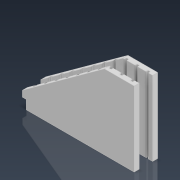
# Autodesk Inventor part: Rising agency
Saved by Autodesk Inventor 2021.1 (Build 251245010, 245A)
## iProperties
Created: 2020-12-20
Part Number: Rising agency
Material: 一般
Document SubType Name: Modeling
Designer: User
Density: 1 g/cm^3
Appearance: 預設
Author: User
Autodesk Inventor part; units mm, degrees
ref_plane "YZ Plane" through (0, 0, 0) normal (1, 0, 0) x (0, 1, 0)
ref_plane "XZ Plane" through (0, 0, 0) normal (0, 1, 0) x (-1, 0, 0)
ref_plane "XY Plane" through (0, 0, 0) normal (0, 0, 1) x (1, 0, 0)
sketch "草圖1" plane through (0, 0, 0) normal (0, 0, 1) x (1, 0, 0)
  line L0 (0, 0) -> (0, 800)
  line L1 (0, 800) -> (-150, 800)
  line L2 (-150, 800) -> (-720, 176.041)
  line L3 (-700, 100) -> (-150, 100)
  line L4 (-150, 100) -> (-150, 0)
  line L5 (-150, 0) -> (0, 0)
  line L6 (-720, 176.041) -> (-720, 146.041)
  line L7 (-720, 146.041) -> (-700, 146.041)
  line L8 (-700, 146.041) -> (-700, 100)
  dimension "d0" = 150
  dimension "d1" = 150
  dimension "d3" = 800
  dimension "d4" = 100
  dimension "d5" = 720
  dimension "d6" = 20
  dimension "d8" = 30
  dimension "d9" = 146.041
  constraints: 18 end point, 5 perpendicular, 2 vertical, 1 horizontal
  measures "d0" distance of L4.end L0.start
  measures "d1" distance of L0.end L1.end
  measures "d3" distance of L0.start L0.end
  measures "d4" distance of L3.end L4.end
  measures "d5" distance between parallel lines of L0 L6
  measures "d6" distance of L6.end L7.end
  measures "d8" distance of L2.end L6.end
  measures "d9" distance between parallel lines of L7 L5
extrude "擠出1" add sketch "草圖1" along normal mid plane 120
sketch "草圖2" plane through (-700, 100, 60) normal (0, -1, 0) x (1, 0, 0)
  line L0 (700, -120) -> (550, -120) construction
  line L1 (550, -120) -> (0, -120) construction
  line L2 (0, -120) -> (0, 0) construction
  line L3 (0, 0) -> (550, 0) construction
  line L4 (550, 0) -> (700, 0) construction
  line L5 (700, 0) -> (700, -120) construction
  line L6 (550, -120) -> (550, 0) construction
  line L7 (-108.104, -26) -> (550, -26)
  line L8 (550, -26) -> (550, -94)
  line L9 (550, -94) -> (-108.104, -94)
  line L10 (-108.104, -94) -> (-108.104, -26)
  point P0 (700, -60)
  point P1 (550, -60)
  dimension "d12" = 68
  constraints: 8 end point, 2 midpoint, 2 parallel, 1 horizontal, 1 perpendicular
  measures "d12" distance of L9.end L7.start
extrude "擠出2" cut sketch "草圖2" against normal through all
sketch "草圖3" plane through (-150, 0, 60) normal (-1, 0, 0) x (0, 0, 1)
  line L0 (-26, 100) -> (-26, 800) projected
  line L1 (-26, 800) -> (0, 800) projected
  line L2 (0, 800) -> (0, 100) projected
  line L3 (0, 100) -> (-26, 100) projected
  line L4 (-94, 800) -> (-26, 800) projected
  line L5 (-120, 800) -> (-94, 800) projected
  line L6 (-120, 100) -> (-120, 800) projected
  line L7 (-94, 100) -> (-120, 100) projected
  line L8 (-94, 800) -> (-94, 100) projected
  line L9 (0, 100) -> (0, 0) projected
  line L10 (0, 0) -> (-120, 0) projected
  line L11 (-120, 0) -> (-120, 100) projected
  circle A0 centre (-60, 50) radius 10
  point P0 (-60, 0)
  point P1 (-60, 0)
  dimension "d15" = 50
  dimension "d16" = 20
  constraints: 1 centre point, 1 midpoint, 1 vertical alignment
  measures "d15" distance from line of L10 A0.centre
  measures "d16" diameter of A0
extrude "擠出3" cut sketch "草圖3" against normal through all contours A0
sketch "草圖4" plane through (-700, 100, 60) normal (0, -1, 0) x (1, 0, 0)
  line L0 (700, -120) -> (550, -120) construction
  line L1 (550, -120) -> (0, -120) construction
  line L2 (0, -120) -> (0, -94) construction
  line L3 (0, -94) -> (550, -94) construction
  line L4 (550, -94) -> (550, -26) construction
  line L5 (550, -26) -> (0, -26) construction
  line L6 (0, -26) -> (0, 0) construction
  line L7 (0, 0) -> (550, 0) construction
  line L8 (550, 0) -> (700, 0) construction
  line L9 (700, 0) -> (700, -120) construction
  line L10 (550, -120) -> (550, -94) construction
  line L11 (550, -26) -> (550, 0) construction
  line L12 (22.5, -16) -> (32.5, -16)
  line L13 (32.5, -16) -> (32.5, -104)
  line L14 (32.5, -104) -> (22.5, -104)
  line L15 (22.5, -104) -> (22.5, -16)
  line L16 (0.5, 0) -> (54.5, 0) construction
  line L17 (54.5, 0) -> (54.5, -120) construction
  line L18 (54.5, -120) -> (0.5, -120) construction
  line L19 (0.5, -120) -> (0.5, 0) construction
  point P0 (700, -60)
  point P1 (27.5, -16)
  point P2 (27.5, 0)
  dimension "d21" = 0.5
  dimension "d22" = 54
  dimension "d23" = 10
  dimension "d24" = 10
  dimension "d25" = 10
  constraints: 16 end point, 4 parallel, 2 collinear, 2 horizontal, 2 midpoint, 2 perpendicular, 1 vertical alignment
  measures "d21" distance between parallel lines of L19 L2
  measures "d22" distance between parallel lines of L17 L19
  measures "d23" distance between parallel lines of L5 L12
  measures "d24" distance between parallel lines of L14 L3
  measures "d25" distance of L13.end L14.end
extrude "擠出4" cut sketch "草圖4" against normal blind 911.5
pattern_linear "矩形陣列1" count 10 spacing 55 along (1, 0, 0) of "擠出4"
sketch "草圖5" plane through (0, 0, 60) normal (0, 0, 1) x (1, 0, 0)
  line L0 (0, 800) -> (0, 0) projected
  line L1 (0, 0) -> (-150, 0) projected
  line L2 (-150, 0) -> (-150, 100) projected
  line L3 (-150, 100) -> (-700, 100) projected
  line L4 (-700, 100) -> (-700, 146.041) projected
  line L5 (-700, 146.041) -> (-720, 146.041) projected
  line L6 (-720, 146.041) -> (-720, 176.041) projected
  line L7 (-720, 176.041) -> (-150, 800) projected
  line L8 (-150, 800) -> (0, 800) projected
  line L9 (-150, 100) -> (-150, 800) projected
  line L10 (-150, 100) -> (-150, 800)
  constraints: 2 end point, 1 collinear
extrude "擠出5" cut sketch "草圖5" against normal through all contours L0 L1 L2 L9 L8
sketch "草圖6" plane through (0, 0, 60) normal (0, 0, 1) x (1, 0, 0)
  line L0 (-150, 800) -> (-150, 100) projected
  line L1 (-150, 100) -> (-700, 100) projected
  line L2 (-700, 100) -> (-700, 146.041) projected
  line L3 (-700, 146.041) -> (-720, 146.041) projected
  line L4 (-720, 146.041) -> (-720, 176.041) projected
  line L5 (-720, 176.041) -> (-150, 800) projected
  line L6 (-720, 176.041) -> (-150, 590)
  line L7 (-150, 100) -> (-150, 800) projected
  point P0 (0, 0)
  point P1 (-150, 590)
  dimension "d33" = 210
  constraints: 2 end point, 1 point on line
  measures "d33" distance of L0.start L6.end
extrude "擠出6" cut sketch "草圖6" against normal through all contours L0 L6 L5
sketch "草圖7" plane through (0, 0, 60) normal (0, 0, 1) x (1, 0, 0)
  line L0 (-720, 146.041) -> (-720, 176.041) projected
  line L1 (-720, 176.041) -> (-150, 590) projected
  line L2 (-150, 590) -> (-150, 100) projected
  line L3 (-150, 100) -> (-700, 100) projected
  line L4 (-700, 100) -> (-700, 146.041) projected
  line L5 (-700, 146.041) -> (-720, 146.041) projected
  line L6 (-301.4643, 480) -> (-150, 480)
  point P0 (0, 0)
  dimension "d36" = 380
  constraints: 2 end point, 2 point on line, 1 horizontal
  measures "d36" distance between parallel lines of L3 L6
extrude "擠出7" cut sketch "草圖7" against normal through all contours L1 L2 L6
